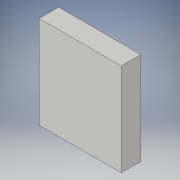
# Autodesk Inventor part: Convex Organ Bank Sensor Slot
Saved by Autodesk Inventor 2019 (Build 230136000, 136)
## iProperties
Created: 2021-02-18
Part Number: Convex Organ Bank Sensor Slot
Material: Generic
Document SubType Name: Modeling
Designer: Eric
Density: 1 g/cm^3
Appearance: Default
Author: Eric
Autodesk Inventor part; units mm, degrees
ref_plane "YZ Plane" through (0, 0, 0) normal (1, 0, 0) x (0, 1, 0)
ref_plane "XZ Plane" through (0, 0, 0) normal (0, 1, 0) x (-1, 0, 0)
ref_plane "XY Plane" through (0, 0, 0) normal (0, 0, 1) x (1, 0, 0)
sketch "Sketch1" plane through (0, 0, 0) normal (0, 0, 1) x (1, 0, 0)
  line L0 (6, -6) -> (36, -6) construction
  line L1 (36, -6) -> (36, -47.4) construction
  line L2 (36, -47.4) -> (6, -47.4) construction
  line L3 (6, -47.4) -> (6, -6) construction
  line L4 (0, 0) -> (42, 0)
  line L5 (42, 0) -> (42, -47.4)
  line L6 (42, -47.4) -> (0, -47.4)
  line L7 (0, -47.4) -> (0, 0)
  dimension "d0" = 30
  dimension "d1" = 41.4
  dimension "d2" = 6
  dimension "d3" = 6
  dimension "d4" = 6
  constraints: 16 end point, 4 horizontal, 4 vertical, 1 collinear
  measures "d0" distance of L1.end L2.end
  measures "d1" distance of L0.end L1.end
  measures "d2" distance between parallel lines of L4 L0
  measures "d3" distance between parallel lines of L7 L3
  measures "d4" distance between parallel lines of L5 L1
extrude "Extrusion1" add sketch "Sketch1" along normal blind 10
body "Solid1"
